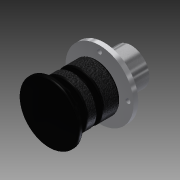
# Autodesk Inventor part: Motor
Saved by Autodesk Inventor 2014 SP1 (Build 180222100, 222)
## iProperties
Created: 2015-03-16
Part Number: Motor
Material: Generic
Document SubType Name: Modeling
Designer: david
Density: 1 g/cm^3
Appearance: Default
Motor_WheelInterface_Diameter: 30,000 mm
Motor_WheelInterface_Length: 27,000 mm
Motor_FasteningHole_DistanceToCenter: 18,000 mm
Author: david
Autodesk Inventor part; units mm, degrees
ref_plane "YZ Plane" through (0, 0, 0) normal (1, 0, 0) x (0, 1, 0)
ref_plane "XZ Plane" through (0, 0, 0) normal (0, 1, 0) x (-1, 0, 0)
ref_plane "XY Plane" through (0, 0, 0) normal (0, 0, 1) x (1, 0, 0)
sketch "BodySketch" plane through (0, 0, 0) normal (1, 0, 0) x (0, 1, 0)
  line L0 (0, 17.5) -> (15, 17.5)
  line L1 (11.5, -34.5) -> (0, -34.5)
  line L2 (0, -34.5) -> (0, 17.5)
  line L3 (15, 1.5) -> (11, 1.5)
  line L4 (11, 1.5) -> (11, -1.5)
  line L5 (11, -1.5) -> (15, -1.5)
  line L6 (15, -1.5) -> (15, -12.5)
  line L7 (0, 0) -> (26.3241, 0) construction
  line L8 (0, 25.0354) -> (0, 0) construction
  line L9 (15, 17.5) -> (19, 17.5)
  line L10 (19, 17.5) -> (19, 14.5)
  line L11 (19, 14.5) -> (15, 14.5)
  line L12 (15, 14.5) -> (15, 17.5) construction
  line L13 (15, 11.5) -> (11, 11.5)
  line L14 (11, 11.5) -> (11, 8.5)
  line L15 (11, 8.5) -> (15, 8.5)
  line L16 (15, 14.5) -> (15, 11.5)
  line L17 (15, 8.5) -> (15, 1.5)
  line L18 (15, -12.5) -> (10, -12.5)
  line L19 (10, -14.5) -> (21.5, -14.5)
  line L20 (21.5, -14.5) -> (21.5, -17.5)
  line L21 (21.5, -17.5) -> (11.5, -17.5)
  line L22 (11.5, -22.5) -> (9.5, -22.5)
  line L23 (9.5, -22.5) -> (9.5, -24.5)
  line L24 (9.5, -24.5) -> (11.5, -24.5)
  line L25 (10, -12.5) -> (10, -14.5)
  line L26 (11.5, -17.5) -> (11.5, -22.5)
  line L27 (11.5, -24.5) -> (11.5, -34.5)
  dimension "Motor_Body_Length" = 52
  dimension "Motor_Body_Belt_Width" = 3
  dimension "Motor_Body_Crown_Height" = 3
  dimension "d14" = 15
  dimension "d15" = 19
  dimension "d16" = 11
  dimension "d17" = 11
  dimension "d18" = 7
  dimension "d19" = 10
  dimension "d20" = 21.5
  dimension "d21" = 11.5
  dimension "d22" = 2
  dimension "d23" = 3
  dimension "d24" = 2
  dimension "d26" = 5
  dimension "d27" = 2
  dimension "d36" = 27
  constraints: 56 end point, 12 perpendicular, 10 parallel, 7 collinear, 7 horizontal, 1 other
  measures "Motor_Body_Length" distance between parallel lines of L1 L0
  measures "Motor_Body_Belt_Width" distance between parallel lines of L5 L3
  measures "Motor_Body_Crown_Height" distance between parallel lines of L0 L11
  measures "d14" distance between parallel lines of L8 L17
  measures "d15" distance between parallel lines of L8 L10
  measures "d16" distance between parallel lines of L8 L14
  measures "d17" distance of L5.end L6.end
  measures "d18" distance of L15.end L3.start
  measures "d19" distance between parallel lines of L2 L25
  measures "d20" distance between parallel lines of L2 L20
  measures "d21" distance between parallel lines of L2 L26
  measures "d22" distance between parallel lines of L27 L23
  measures "d23" distance between parallel lines of L21 L19
  measures "d24" distance between parallel lines of L24 L22
  measures "d26" distance of L21.end L22.start
  measures "d27" distance between parallel lines of L19 L18
  measures "d36" distance between parallel lines of L11 L18
revolve "Body" add sketch "BodySketch" angle 360 about axis through (0, 0, 25.0354) along (0, 0, -1)
fillet "Fillet1" radius 1 7 edges at (0, -19, 14.5) (0, -15, 1.5) (0, -15, -1.5) (0, -15, -12.5) (0, -19, 17.5) (0, -15, 11.5) (0, -15, 8.5)
sketch "FasteningHoleSketch" plane through (0, 0, -17.5) normal (0, 0, -1) x (-1, 0, 0)
  circle A0 centre (0, 0) radius 11.5 projected
  circle A1 centre (0, 0) radius 21.5 projected
  circle A2 centre (0, 18) radius 1.5
  line L0 (0, 0) -> (0, 24.6979) construction
  circle A3 centre (18, 0) radius 1.5
  circle A4 centre (0, -18) radius 1.5
  circle A5 centre (-18, 0) radius 1.5
  dimension "Motor_FasteningHole_Size" = 3
  dimension "Motor_FasteningHole_DistanceToBorder" = 2
  dimension "d32" = 360
  constraints: 4 centre point, 2 end point, 1 point on line, 1 vertical, 9 other
  measures "Motor_FasteningHole_Size" diameter of A2
extrude "FasteningHole" cut sketch "FasteningHoleSketch" against normal up to surface (3 mm away) contours A2 | A3 | A4 | A5
equation "\"d14\" = 0.5 * Motor_WheelInterface_Diameter"
equation "\"d36\" = Motor_WheelInterface_Length"
equation "\"Motor_WheelInterface_Diameter\" = 30"
equation "\"Motor_WheelInterface_Length\" = 27"
equation "\"Motor_FasteningHole_DistanceToCenter\" = 18"
body "Solid2"
